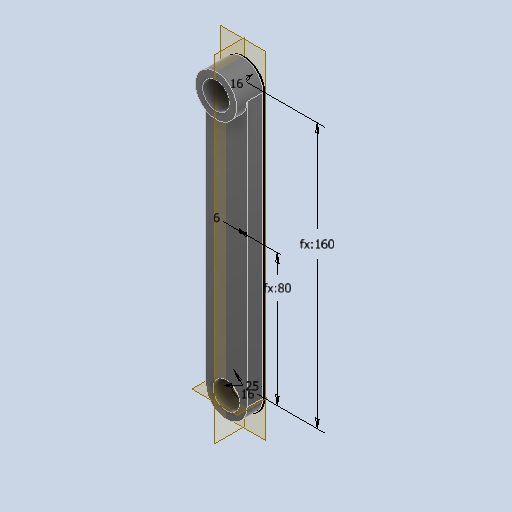
# Autodesk Inventor part: ParallelSystem_ProximalPart_SupportLink
Saved by Autodesk Inventor 2024 (Build 280153000, 153)
## iProperties
Created: 2022-07-18
Part Number: ParallelSystem_ProximalPart_SupportLink
Material: PBT-Kunststoff
Document SubType Name: Modeling
Designer: alexw
Density: 1.31 g/cm^3
Appearance: Glatt - Schwarz
Mass: 55.8894 g
Surface Area: 138.626 cm^2
Volume: 42.6636 cm^3
d7: 5,000 mm
d9: 6,000 mm
d37: 30,000 mm
d44: 12,000 mm
ParallelLink_BearingStep_Height: 10,000 mm
Link_Thickness: 10,000 mm
LinkThickness: 10,000 mm
Anlaufscheibe_Thickness: 1,000 mm
Rillenkugellager_Flanschdicke: 1,100 mm
SupportLink_Step_Thickness: 6,300 mm
Author: alexw
Autodesk Inventor part; units mm, degrees
sketch "Skizze5" plane through (0, 0, 0) normal (0, 0, 1) x (1, 0, 0)
  circle A0 centre (0, 0) radius 12.5
  circle A1 centre (0, 0) radius 8
  circle A2 centre (0, 160) radius 12.5
  circle A3 centre (0, 160) radius 8
  line L0 (0, 0) -> (0, 160) construction
  line L1 (-12.5, 0) -> (-12.5, 160)
  line L2 (12.5, 0) -> (12.5, 160)
  circle A4 centre (0, 80) radius 3
  dimension "d98" = 25
  dimension "d99" = 16
  dimension "d100" = 160
  dimension "d110" = 16
  dimension "d116" = 6
  dimension "d117" = 80
  constraints: 6 end point, 5 centre point, 4 point on circle, 4 tangent, 3 coincident, 1 equal radius, 1 midpoint, 1 vertical
  measures "d98" diameter of A0
  measures "d99" diameter of A1
  measures "d100" distance of L0.start L0.end
  measures "d110" diameter of A3
  measures "d116" diameter of A4
  measures "d117" distance of A4.centre point (0, 0)
extrude "Extrusion8" add sketch "Skizze5" along normal blind 10 contours A0 | A0 L1 A2 L2 | A2 | A4
extrude "Extrusion12" add sketch "Skizze5" along normal blind 6.3 from surface at 10 contours A2
chamfer "Fase1" distance 0.5 angle 45 4 edges at (-12.5, 80, 0) (0, -12.5, 0) (12.5, 80, 0) (0, 172.5, 0)
equation "\"Anlaufscheibe_Thickness\" = 1"
equation "\"BaseFrame_InnerWidth\" = 83"
equation "\"Rillenkugellager_Flanschdicke\" = 1.1"
